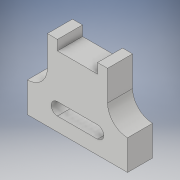
# Autodesk Inventor part: P2-5
Saved by Autodesk Inventor 2017 (Build 210142000, 142)
## iProperties
Created: 2017-02-09
Part Number: P2-5
Material: Generic
Document SubType Name: Modeling
Designer: Schaffel
Density: 1 g/cm^3
Appearance: Default
Author: Schaffel
Autodesk Inventor part; units mm, degrees
ref_plane "YZ Plane" through (0, 0, 0) normal (1, 0, 0) x (0, 1, 0)
ref_plane "XZ Plane" through (0, 0, 0) normal (0, 1, 0) x (-1, 0, 0)
ref_plane "XY Plane" through (0, 0, 0) normal (0, 0, 1) x (1, 0, 0)
sketch "Sketch1" plane through (0, 0, 0) normal (0, 0, 1) x (1, 0, 0)
  line L0 (0, 38.1) -> (0, 0)
  line L1 (0, 0) -> (127, 0)
  line L2 (127, 0) -> (127, 38.1)
  arc A0 (0, 38.1) -> (25.4, 63.5) centre (0, 63.5) ccw
  arc A1 (101.6, 63.5) -> (127, 38.1) centre (127, 63.5) ccw
  line L3 (25.4, 101.6) -> (25.4, 63.5)
  line L4 (25.4, 101.6) -> (38.1, 101.6)
  line L5 (38.1, 101.6) -> (38.1, 88.9)
  line L6 (38.1, 88.9) -> (88.9, 88.9)
  line L7 (88.9, 88.9) -> (88.9, 101.6)
  line L8 (88.9, 101.6) -> (101.6, 101.6)
  line L9 (101.6, 101.6) -> (101.6, 63.5)
  arc A2 (38.1, 33.3375) -> (38.1, 17.4625) centre (38.1, 25.4) ccw
  arc A3 (88.9, 17.4625) -> (88.9, 33.3375) centre (88.9, 25.4) ccw
  line L10 (88.9, 33.3375) -> (38.1, 33.3375)
  line L11 (38.1, 17.4625) -> (88.9, 17.4625)
  constraints: 24 end point, 8 point on circle, 6 perpendicular, 4 centre point, 2 horizontal, 2 point on line, 2 vertical, 1 parallel
extrude "Extrusion1" add sketch "Sketch1" along normal blind 31.75
body "Solid1"
